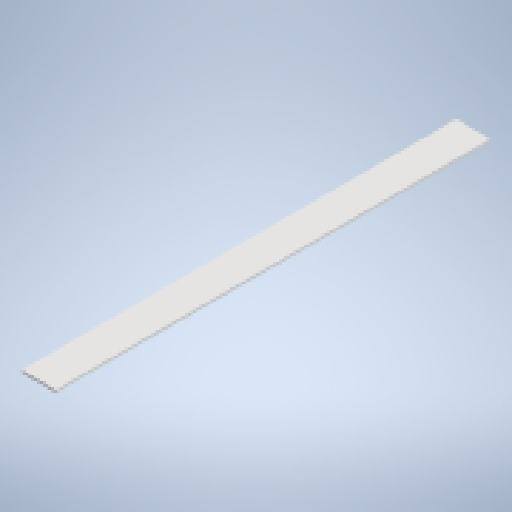
# Autodesk Inventor part: GBK bottom 0128
Saved by Autodesk Inventor 2026 (Build 300175000, 175)
## iProperties
Created: 2026-05-19
Part Number: GBK bottom 0128
Material: Steel
Document SubType Name: Sheet Metal
Designer: admin
Mass: 3778.05 g
Surface Area: 2081.92 cm^2
Volume: 481.28 cm^3
Density: 7.85 g/cm^3
Flat Pattern Width: 6.4 cm
Flat Pattern Length: 81.6 cm
Flat Pattern Area: 522.24 cm^2
Sheet Metal Rule: По умолчанию_мм
Sheet Metal Width: 64,000 мм
Sheet Metal Length: 816,000 мм
Sheet Metal Area: 52224,000 мм^2
Appearance: Default
Author: user
Autodesk Inventor part; units mm, degrees
ref_plane "YZ Plane" through (0, 0, 0) normal (1, 0, 0) x (0, 1, 0)
ref_plane "XZ Plane" through (0, 0, 0) normal (0, 1, 0) x (-1, 0, 0)
ref_plane "XY Plane" through (0, 0, 0) normal (0, 0, 1) x (1, 0, 0)
sketch "Эскиз1" plane through (0, 0, 0) normal (0, 1, 0) x (-1, 0, 0)
  line L0 (-32, 408) -> (32, 408)
  line L1 (32, 408) -> (32, -408)
  line L2 (32, -408) -> (-32, -408)
  line L3 (-32, -408) -> (-32, 408)
  line L4 (-32, 408) -> (32, -408) construction
  line L5 (32, 408) -> (-32, -408) construction
  point P0 (0, 0)
  dimension "d0" = 64
  dimension "d1" = 816
  measures "d0" distance of L1.end L2.end
  measures "d1" distance of L0.end L1.end
extrude "Пластина1" add sketch "Эскиз1" along normal blind 5
equation "\"d2\" = Толщина"
equation "\"Радиус_гибки\" = Толщина"
equation "\"Ширина_просечки\" = Толщина"
equation "\"Глубина_просечки\" = 0.5 * Толщина"
equation "\"Радиус_перехода\" = Радиус_гибки"
equation "\"Радиус_Якоби\" = Радиус_гибки"
equation "\"Размер_зазора\" = Толщина"
equation "\"Толщина\" = 5"
